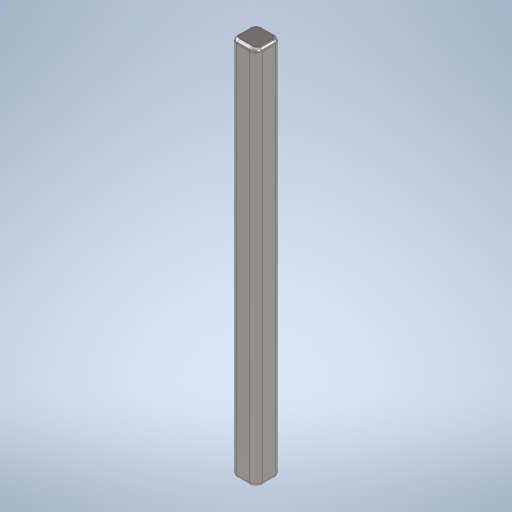
# Autodesk Inventor part: wedgea
Saved by Autodesk Inventor 2023 (Build 270158000, 158)
## iProperties
Created: 2022-05-23
Part Number: wedgea
Material: Stainless Steel
Document SubType Name: Modeling
Designer: aaron
Density: 8 g/cm^3
Appearance: Semi-Polished
Author: aaron
Autodesk Inventor part; units mm, degrees
ref_plane "YZ Plane" through (0, 0, 0) normal (1, 0, 0) x (0, 1, 0)
ref_plane "XZ Plane" through (0, 0, 0) normal (0, 1, 0) x (-1, 0, 0)
ref_plane "XY Plane" through (0, 0, 0) normal (0, 0, 1) x (1, 0, 0)
sketch "Sketch1" plane through (0, 0, 0) normal (0, 1, 0) x (-1, 0, 0)
  line L0 (-3.175, -3.175) -> (3.175, -3.175)
  line L1 (3.175, -3.175) -> (3.175, 3.175)
  line L2 (3.175, 3.175) -> (-3.175, 3.175)
  line L3 (-3.175, 3.175) -> (-3.175, -3.175)
  line L4 (-3.175, -3.175) -> (3.175, 3.175) construction
  line L5 (3.175, -3.175) -> (-3.175, 3.175) construction
  point P0 (0, 0)
  dimension "d2" = 6.35
  dimension "d3" = 6.35
  constraints: 12 end point, 2 midpoint, 2 parallel, 1 horizontal, 1 perpendicular
  measures "d2" distance of L2.end L1.end
  measures "d3" distance of L1.end L0.end
extrude "Extrusion1" add sketch "Sketch1" along normal blind 93.98
fillet "Fillet1" radius 1.5875 4 edges at (3.175, 46.99, 3.175) (3.175, 46.99, -3.175) (-3.175, 46.99, -3.175) (-3.175, 46.99, 3.175)
fillet "Fillet2" radius 0.7937 16 edges at (3.175, 0, 0) (2.71, 0, -2.71) (0, 0, -3.175) (-2.71, 0, -2.71) (-3.175, 0, 0) (-2.71, 0, 2.71) (0, 0, 3.175) (2.71, 0, 2.71) (0, 93.98, 3.175) (-2.71, 93.98, 2.71) (-3.175, 93.98, 0) (-2.71, 93.98, -2.71) (0, 93.98, -3.175) (2.71, 93.98, -2.71) (3.175, 93.98, 0) (2.71, 93.98, 2.71)
body "Solid1"
